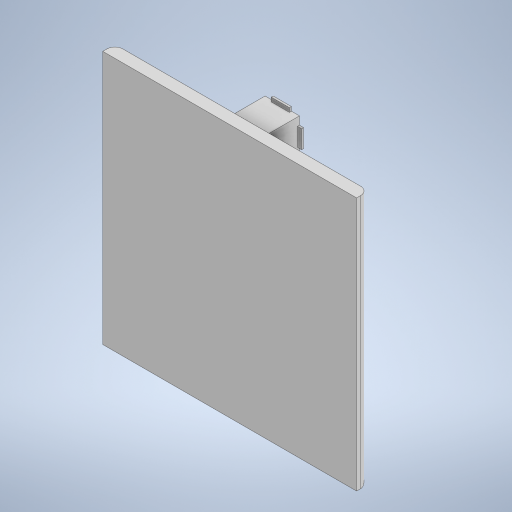
# Autodesk Inventor part: GroundV11
Saved by Autodesk Inventor 2024 (Build 280153000, 153)
## iProperties
Created: 2024-01-02
Part Number: GroundV11
Material: Generisch
Document SubType Name: Modeling
Designer: chris
Density: 1 g/cm^3
Appearance: Vorgabe
Author: chris
Autodesk Inventor part; units mm, degrees
ref_plane "YZ Plane" through (0, 0, 0) normal (1, 0, 0) x (0, 1, 0)
ref_plane "XZ Plane" through (0, 0, 0) normal (0, 1, 0) x (-1, 0, 0)
ref_plane "XY Plane" through (0, 0, 0) normal (0, 0, 1) x (1, 0, 0)
sketch "Skizze1" plane through (0, 0, 0) normal (0, 1, 0) x (-1, 0, 0)
  line L0 (-31.35, 31.35) -> (31.35, 31.35)
  line L1 (31.35, 31.35) -> (31.35, -31.35)
  line L2 (31.35, -31.35) -> (-31.35, -31.35)
  line L3 (-31.35, -31.35) -> (-31.35, 31.35)
  line L4 (-31.35, 31.35) -> (31.35, -31.35) construction
  line L5 (31.35, 31.35) -> (-31.35, -31.35) construction
  point P0 (0, 0)
  dimension "d0" = 62.7
  dimension "d1" = 62.7
  constraints: 12 end point, 2 midpoint, 2 parallel, 1 horizontal, 1 perpendicular
  measures "d0" distance of L1.end L2.end
  measures "d1" distance of L0.end L1.end
extrude "Extrusion1" add sketch "Skizze1" along normal mid plane 3
sketch "Skizze2" plane through (0, 1.5, 0) normal (0, 1, 0) x (1, 0, 0)
  line L0 (-31.35, -31.35) -> (31.35, -31.35) construction
  line L1 (0, -31.35) -> (0, 0) construction
  line L2 (4.25, -28.85) -> (-4.25, -28.85)
  line L3 (-4.25, -28.85) -> (-4.25, -20.35)
  line L4 (-4.25, -20.35) -> (4.25, -20.35)
  line L5 (4.25, -20.35) -> (4.25, -28.85)
  dimension "d6" = 2.5
  dimension "d7" = 8.5
  dimension "d9" = 4.25
  dimension "d10" = 4.25
  constraints: 10 end point, 2 parallel, 1 horizontal, 1 midpoint, 1 perpendicular, 1 vertical
  measures "d6" distance between parallel lines of L0 L2
  measures "d7" distance between parallel lines of L2 L4
  measures "d9" distance between parallel lines of L1 L3
  measures "d10" distance between parallel lines of L5 L1
extrude "Extrusion2" add sketch "Skizze2" along normal blind 10
sketch "Skizze3" plane through (0, 11.5, 0) normal (0, 1, 0) x (1, 0, 0)
  line L0 (-4.25, -28.85) -> (-4.25, -20.35) projected
  line L1 (4.25, -20.35) -> (4.25, -28.85) projected
  line L2 (-4.25, -28.85) -> (4.25, -28.85)
  line L3 (-4.25, -26.85) -> (-5.25, -26.85)
  line L4 (4.25, -26.85) -> (5.25, -26.85)
  line L5 (-4.25, -20.35) -> (4.25, -20.35) projected
  line L6 (-2.25, -20.35) -> (-2.25, -19.35)
  line L7 (-2.25, -19.35) -> (2.25, -19.35)
  line L8 (2.25, -19.35) -> (2.25, -20.35)
  line L9 (-2.25, -28.85) -> (-2.25, -29.85)
  line L10 (-2.25, -29.85) -> (2.25, -29.85)
  line L11 (2.25, -29.85) -> (2.25, -28.85)
  line L12 (5.25, -26.85) -> (5.25, -22.35)
  line L13 (5.25, -22.35) -> (4.25, -22.35)
  line L14 (-5.25, -26.85) -> (-5.25, -22.35)
  line L15 (-5.25, -22.35) -> (-4.25, -22.35)
  point P0 (0, 0)
  dimension "d18" = 1
  dimension "d19" = 1
  dimension "d21" = 1
  dimension "d22" = 1
  dimension "d23" = 2
  dimension "d24" = 2
  dimension "d25" = 2
  dimension "d26" = 2
  dimension "d27" = 2
  dimension "d28" = 2
  dimension "d29" = 2
  constraints: 26 end point, 10 point on line, 7 perpendicular, 3 vertical, 2 horizontal
  measures "d18" distance of L3.start L3.end
  measures "d19" distance of L4.start L4.end
  measures "d21" distance of L6.start L6.end
  measures "d22" distance of L9.start L9.end
  measures "d23" distance between parallel lines of L9 L0
  measures "d24" distance between parallel lines of L11 L1
  measures "d25" distance between parallel lines of L4 L2
  measures "d26" distance between parallel lines of L5 L13
  measures "d27" distance between parallel lines of L8 L1
  measures "d28" distance between parallel lines of L6 L0
  measures "d29" distance between parallel lines of L5 L15
extrude "Extrusion3" add sketch "Skizze3" against normal blind 0.5 contours L3 L14 L15 L0 | L2 L11 L10 L9 | L6 L7 L8 L5 | L1 L13 L12 L4
fillet "Rundung1" radius 2 3 edges at (-31.35, 1.5, 0) (0, 1.5, -31.35) (31.35, 1.5, 0)
